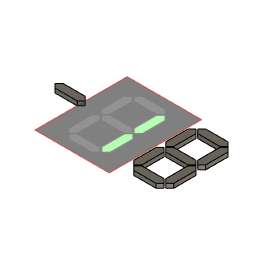
2023_02_18_Digit Clock Mesh v4 (Autodesk Fusion 360 design; units mm, degrees)
Autodesk Fusion 360 part; units mm, degrees
sketch "Sketch1" plane through (0, 0, 0) normal (0, 0, 1) x (1, 0, 0)
  line L0 (2.6688, 1.1143) -> (4.5534, 1.1143) construction
  line L1 (4.5534, 1.1143) -> (4.5534, 6.3417)
  line L2 (4.5534, 6.3417) -> (2.6688, 6.3417) construction
  line L3 (2.6688, 6.3417) -> (2.6688, 1.1143)
  line L4 (3.6111, 6.3417) -> (3.6111, 7.2772) construction
  line L5 (3.6111, 7.2772) -> (2.6688, 6.3417)
  line L6 (3.6111, 7.2772) -> (4.5534, 6.3417)
  line L7 (3.6111, 1.1143) -> (3.6111, 0.1788) construction
  line L8 (3.6111, 0.1788) -> (4.5534, 1.1143)
  line L9 (2.6688, 1.1143) -> (3.6111, 0.1788)
  constraint horizontal L0
  constraint vertical L1
  constraint horizontal L2
  constraint vertical L3
  constraint midpoint L2 L4.start
  constraint perpendicular L2 L4
  constraint midpoint L0 L7.start
  constraint perpendicular L0 L7
  constraint equal L4 L7
extrude "Extrude1" add sketch "Sketch1" along normal blind 1 makes body 1
move_body "Move1" bodies 1 to x (0, 1, 0) y (-1, 0, 0) z (0, 0, 1) at (4.1788, -0.1863, 0)
move_body "Move2" bodies 1 to x (1, 0, 0) y (0, 1, 0) z (0, 0, 1) at (-0.7301, -3.4436, 0)
copy_body "CopyPasteBodies1" bodies 1 makes body 2
move_body "Move3" bodies 2 to x (0, 1, 0) y (-1, 0, 0) z (0, 0, 1) at (-3.8472, 3.8097, 0)
copy_body "CopyPasteBodies2" bodies 1 makes body 3
move_body "Move4" bodies 3 to x (0, -1, 0) y (1, 0, 0) z (0, 0, 1) at (-3.8097, -3.8472, 0)
copy_body "CopyPasteBodies3" bodies 2 3 makes body 4 makes body 5
move_body "Move5" bodies 4 5 to x (1, 0, 0) y (0, 1, 0) z (0, 0, 1) at (7.0983, 0, 0)
copy_body "CopyPasteBodies4" bodies 1 makes body 6
move_body "Move6" bodies 6 to x (1, 0, 0) y (0, 1, 0) z (0, 0, 1) at (0, -7.0983, 0)
copy_body "CopyPasteBodies5" bodies 1 makes body 7
move_body "Move7" bodies 7 to x (1, 0, 0) y (0, 1, 0) z (0, 0, 1) at (0, 7.0983, 0)
copy_body "CopyPasteBodies6" bodies 7 4 2 3 6 1 5 makes body 8 makes body 9 makes body 10 makes body 11 makes body 12 makes body 13 makes body 14
move_body "Move8" bodies 8 9 10 11 12 13 14 to x (1, 0, 0) y (0, 1, 0) z (0, 0, 1) at (15, 0, 0)
move_body "Move9" bodies 10 to x (1, 0, 0) y (0, 1, 0) z (0, 0, 1) at (-0.2, 0.2, 0)
move_body "Move10" bodies 9 to x (1, 0, 0) y (0, 1, 0) z (0, 0, 1) at (0.2, 0.2, 0)
move_body "Move11" bodies 14 to x (1, 0, 0) y (0, 1, 0) z (0, 0, 1) at (0.2, -0.2, 0)
move_body "Move12" bodies 11 to x (1, 0, 0) y (0, 1, 0) z (0, 0, 1) at (-0.2, -0.2, 0)
move_body "Move13" bodies 8 to x (1, 0, 0) y (0, 1, 0) z (0, 0, 1) at (0, 0.4, 0)
move_body "Move14" bodies 12 to x (1, 0, 0) y (0, 1, 0) z (0, 0, 1) at (0, -0.4, 0)
copy_body "CopyPasteBodies7" bodies 1 makes body 15
move_body "Move15" bodies 15 to x (1, 0, 0) y (0, 1, 0) z (0, 0, 1) at (-11, 0, 0)
named bodies: "Digit Piece"
